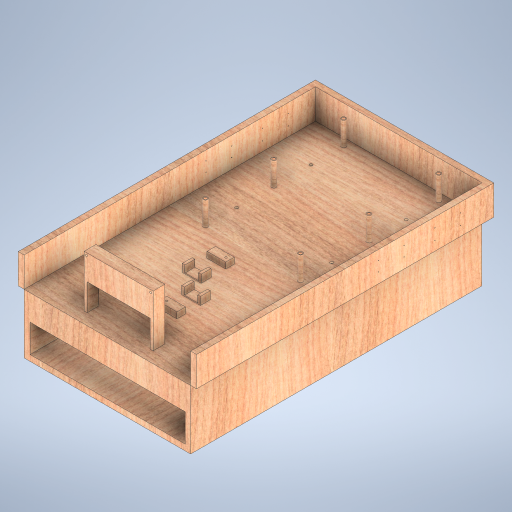
# Autodesk Inventor part: box
Saved by Autodesk Inventor 2024.3 (Build 283343000, 343)
## iProperties
Created: 2024-12-06
Part Number: box
Material: Wood (Birch)
Document SubType Name: Modeling
Designer: PRE 7730
Density: 0.55 g/cm^3
Appearance: Birch - Natural Polished
Author: PRE 7730
Autodesk Inventor part; units mm, degrees
ref_plane "YZ Plane" through (0, 0, 0) normal (1, 0, 0) x (0, 1, 0)
ref_plane "XZ Plane" through (0, 0, 0) normal (0, 1, 0) x (-1, 0, 0)
ref_plane "XY Plane" through (0, 0, 0) normal (0, 0, 1) x (1, 0, 0)
sketch "Sketch2" plane through (0, 0, 0) normal (0, 1, 0) x (-1, 0, 0)
  line L0 (14.4657, 20.7206) -> (-285.5343, 20.7206)
  line L1 (-285.5343, 20.7206) -> (-285.5343, -479.2794)
  line L2 (-285.5343, -479.2794) -> (14.4657, -479.2794)
  line L3 (14.4657, -479.2794) -> (14.4657, 20.7206)
  line L4 (-275.5343, 10.7206) -> (-275.5343, -469.2794)
  line L5 (-275.5343, -469.2794) -> (4.4657, -469.2794)
  line L6 (4.4657, -469.2794) -> (4.4657, 10.7206)
  line L7 (4.4657, 10.7206) -> (4.4657, 20.7206)
  line L8 (-275.5343, 10.7206) -> (-275.5343, 20.7206)
  point P0 (0, 0)
  dimension "d5" = 300
  dimension "d6" = 500
  dimension "d7" = 10
  constraints: 18 end point, 3 parallel, 3 perpendicular, 2 point on line, 1 horizontal, 2 other
  measures "d5" distance of L2.end L1.end
  measures "d6" distance of L1.end L0.end
  measures "d7" distance between parallel lines of L3 L6
extrude "Extrusion2" add sketch "Sketch2" against normal blind 100 contours L7 L6 L5 L4 L8 L0
extrude "Extrusion3" add sketch "Sketch2" along normal blind 50 contours L3 L2 L1 L0 L8 L4 L5 L6 L7
sketch "Sketch3" plane through (0, 0, 0) normal (0, 1, 0) x (1, 0, 0)
  point P0 (0, 0)
sketch "Sketch4" plane through (0, 0, 0) normal (0, 1, 0) x (1, 0, 0)
  line L0 (-4.4657, 469.2794) -> (-4.4657, -20.7206) projected
  line L1 (-4.4657, -20.7206) -> (275.5343, -20.7206) projected
  line L2 (275.5343, -20.7206) -> (275.5343, 469.2794) projected
  line L3 (275.5343, 469.2794) -> (-4.4657, 469.2794) projected
  line L4 (265.5343, 439.2794) -> (165.5343, 439.2794)
  line L5 (165.5343, 439.2794) -> (165.5343, 364.2794)
  line L6 (165.5343, 364.2794) -> (265.5343, 364.2794)
  line L7 (265.5343, 364.2794) -> (265.5343, 439.2794)
  line L8 (-4.4657, 469.2794) -> (275.5343, 469.2794)
  line L9 (-4.4657, 469.2794) -> (275.5343, 469.2794)
  line L10 (135.5343, 469.2794) -> (135.5343, 234.4175)
  line L11 (0, 339.2794) -> (275.5343, 339.2794)
  line L12 (5.5343, 439.2794) -> (105.5343, 439.2794)
  line L13 (105.5343, 439.2794) -> (105.5343, 364.2794)
  line L14 (105.5343, 364.2794) -> (5.5343, 364.2794)
  line L15 (5.5343, 364.2794) -> (5.5343, 439.2794)
  line L16 (265.5343, 239.2794) -> (165.5343, 239.2794)
  line L17 (165.5343, 239.2794) -> (165.5343, 314.2794)
  line L18 (165.5343, 314.2794) -> (265.5343, 314.2794)
  line L19 (265.5343, 314.2794) -> (265.5343, 239.2794)
  line L20 (5.5343, 239.2794) -> (105.5343, 239.2794)
  line L21 (105.5343, 239.2794) -> (105.5343, 314.2794)
  line L22 (105.5343, 314.2794) -> (5.5343, 314.2794)
  line L23 (5.5343, 314.2794) -> (5.5343, 239.2794)
  line L24 (135.5343, 79.3017) -> (167.0343, 79.3017)
  line L25 (167.0343, 79.3017) -> (167.0343, 64.8017)
  line L26 (167.0343, 64.8017) -> (135.5343, 64.8017)
  line L27 (135.5343, 64.8017) -> (135.5343, 79.3017)
  circle A0 centre (142.2843, 72.2017) radius 1.5
  line L28 (135.5343, 120.7409) -> (167.2853, 120.7409)
  line L29 (167.2853, 120.7409) -> (167.2853, 103.9909)
  line L30 (167.2853, 103.9909) -> (135.5343, 103.9909)
  line L31 (135.5343, 103.9909) -> (135.5343, 120.7409)
  line L32 (135.5343, 192.8569) -> (135.5343, 178.3569)
  line L33 (135.5343, 153.6678) -> (135.5343, 136.9178)
  line L34 (103.7833, 136.9178) -> (103.7833, 153.6678)
  line L35 (103.7833, 153.6678) -> (135.5343, 153.6678)
  circle A1 centre (128.7843, 185.4569) radius 1.5
  line L36 (135.5343, 178.3569) -> (104.0343, 178.3569)
  line L37 (104.0343, 178.3569) -> (104.0343, 192.8569)
  line L38 (104.0343, 192.8569) -> (135.5343, 192.8569)
  line L39 (135.5343, 136.9178) -> (103.7833, 136.9178)
  circle A2 centre (55.5343, 401.7794) radius 2.5
  circle A3 centre (215.5343, 401.7794) radius 2.5
  circle A4 centre (55.5343, 276.7794) radius 2.5
  circle A5 centre (215.5343, 276.7794) radius 2.5
  line L40 (275.5343, 469.2794) -> (275.5343, -20.7206) projected
  line L41 (-4.4657, -20.7206) -> (275.5343, -20.7206)
  line L42 (275.5343, -20.7206) -> (275.5343, -10.7206)
  line L43 (-4.4657, -10.7206) -> (-4.4657, -20.7206)
  line L44 (-4.4657, 469.2794) -> (-4.4657, -20.7206) projected
  line L45 (-4.4657, -20.7206) -> (275.5343, -20.7206) projected
  line L46 (275.5343, -20.7206) -> (275.5343, 469.2794) projected
  line L47 (275.5343, 469.2794) -> (-4.4657, 469.2794) projected
  line L48 (77.5343, 18.1016) -> (193.5343, 18.1016)
  line L49 (193.5343, 18.1016) -> (193.5343, -1.8984)
  line L50 (193.5343, -1.8984) -> (77.5343, -1.8984)
  line L51 (77.5343, -1.8984) -> (77.5343, 18.1016)
  circle A6 centre (55.5343, 456.7551) radius 3.75
  circle A7 centre (55.5343, 339.2794) radius 3.75
  circle A8 centre (55.5343, 224.2794) radius 3.75
  circle A9 centre (215.5343, 456.7551) radius 3.75
  circle A10 centre (215.5343, 339.2794) radius 3.75
  circle A11 centre (215.5343, 224.2794) radius 3.75
  circle A12 centre (55.5343, 456.7551) radius 2.5
  circle A13 centre (215.5343, 456.7551) radius 2.5
  circle A14 centre (215.5343, 339.2794) radius 2.5
  circle A15 centre (215.5343, 224.2794) radius 2.5
  circle A16 centre (55.5343, 224.2794) radius 2.5
  circle A17 centre (55.5343, 339.2794) radius 2.5
  point P0 (0, 0)
  point P1 (77.5343, 8.1016)
  dimension "d13" = 100
  dimension "d14" = 75
  dimension "d15" = 30
  dimension "d16" = 10
  dimension "d18" = 25
  dimension "d33" = 31.5
  dimension "d34" = 14.5
  dimension "d35" = 3
  dimension "d36" = 6.75
  dimension "d37" = 7.1
  dimension "d38" = 31.751
  dimension "d39" = 16.75
  dimension "d69" = 5
  dimension "d70" = 37.5
  dimension "d71" = 50
  dimension "d75" = 116
  dimension "d76" = 20
  dimension "d77" = 82
  dimension "d90" = 7.5
  dimension "d91" = 80
  dimension "d92" = 7.5
  dimension "d93" = 80
  dimension "d94" = 7.5
  dimension "d95" = 80
  dimension "d98" = 5
  dimension "d99" = 5
  dimension "d100" = 5
  dimension "d101" = 5
  dimension "d102" = 5
  dimension "d103" = 5
  constraints: 86 end point, 18 centre point, 18 symmetric about line, 9 parallel, 8 perpendicular, 6 coincident, 5 horizontal, 3 point on line, 2 midpoint, 1 vertical, 6 other
  measures "d13" distance of L6.end L5.end
  measures "d14" distance of L5.end L4.end
  measures "d15" distance between parallel lines of L4 L3
  measures "d16" distance between parallel lines of L2 L7
  measures "d18" distance between parallel lines of L11 L6
  measures "d33" distance of L25.end L26.end
  measures "d34" distance of L24.end L25.end
  measures "d35" diameter of A0
  measures "d36" distance from line of L27 A0.centre
  measures "d37" distance from line of L24 A0.centre
  measures "d38" distance of L29.end L30.end
  measures "d39" distance of L28.end L29.end
  measures "d69" diameter of A2
  measures "d70" distance from line of A2.centre L12
  measures "d71" distance from line of L15 A2.centre
  measures "d75" distance of L49.end L50.end
  measures "d76" distance of L48.end L49.end
  measures "d77" distance from line of L0 point (77.534, 8.102)
  measures "d90" diameter of A6
  measures "d91" distance from line of L10 A6.centre
  measures "d92" diameter of A7
  measures "d93" distance from line of L10 A7.centre
  measures "d94" diameter of A8
  measures "d95" distance from line of L10 A8.centre
  measures "d98" diameter of A12
  measures "d99" diameter of A13
  measures "d100" diameter of A14
  measures "d101" diameter of A15
  measures "d102" diameter of A16
  measures "d103" diameter of A17
extrude "Extrusion4" add sketch "Sketch4" along normal blind 10 contours L32 L36 L37 L38
sketch "Sketch5" plane through (-4.4657, -100, 20.7206) normal (0, 0, 1) x (1, 0, 0)
  line L0 (0, 100) -> (0, 0) projected
  line L1 (0, 67.0561) -> (280.9321, 67.0561)
  line L2 (280.9321, 67.0561) -> (280.9321, 0)
  line L3 (280.9321, 0) -> (0, 0)
  line L4 (0, 0) -> (0, 67.0561)
  line L5 (270.9321, 57.0561) -> (10, 57.0561)
  line L6 (10, 57.0561) -> (10, 10)
  line L7 (10, 10) -> (270.9321, 10)
  line L8 (270.9321, 10) -> (270.9321, 57.0561)
  point P0 (4.4657, 100)
  dimension "d24" = 10
  constraints: 16 end point, 4 perpendicular, 1 collinear, 1 horizontal, 1 point on line, 3 other
  measures "d24" distance between parallel lines of L1 L5
extrude "Extrusion5" cut sketch "Sketch5" against normal through all contours L8 L7 L6 L5
extrude "Extrusion6" add sketch "Sketch4" along normal blind 10 contours L33 L39 L34 L35
extrude "Extrusion7" add sketch "Sketch4" along normal blind 13 contours L28 L29 L30 L31 | L33 L39 L34 L35
extrude "Extrusion8" add sketch "Sketch4" along normal blind 10 contours L24 L25 L26 L27
sketch "Sketch6" plane through (0, 13, 0) normal (0, 1, 0) x (1, 0, 0)
  line L0 (104.0343, 192.8569) -> (135.5343, 192.8569) projected
  line L1 (135.5343, 192.8569) -> (135.5343, 178.3569) projected
  line L2 (135.5343, 178.3569) -> (104.0343, 178.3569) projected
  line L3 (104.0343, 178.3569) -> (104.0343, 192.8569) projected
  line L4 (-4.4657, 469.2794) -> (-4.4657, -20.7206) projected
  line L5 (-4.4657, -20.7206) -> (275.5343, -20.7206) projected
  line L6 (275.5343, -20.7206) -> (275.5343, 469.2794) projected
  line L7 (275.5343, 469.2794) -> (-4.4657, 469.2794) projected
  line L8 (103.7833, 153.6678) -> (135.5343, 153.6678) projected
  line L9 (135.5343, 153.6678) -> (135.5343, 136.9178) projected
  line L10 (135.5343, 136.9178) -> (103.7833, 136.9178) projected
  line L11 (103.7833, 136.9178) -> (103.7833, 153.6678) projected
  line L12 (135.5343, 103.9909) -> (135.5343, 120.7409) projected
  line L13 (135.5343, 120.7409) -> (167.2853, 120.7409) projected
  line L14 (167.2853, 120.7409) -> (167.2853, 103.9909) projected
  line L15 (167.2853, 103.9909) -> (135.5343, 103.9909) projected
  line L16 (135.5343, 64.8017) -> (135.5343, 79.3017) projected
  line L17 (135.5343, 79.3017) -> (167.0343, 79.3017) projected
  line L18 (167.0343, 79.3017) -> (167.0343, 64.8017) projected
  line L19 (167.0343, 64.8017) -> (135.5343, 64.8017) projected
  line L20 (103.7833, 153.6678) -> (135.5343, 153.6678)
  line L21 (135.5343, 153.6678) -> (135.5343, 136.9178)
  line L22 (135.5343, 136.9178) -> (103.7833, 136.9178)
  line L23 (103.7833, 136.9178) -> (103.7833, 153.6678)
  line L24 (108.4088, 153.6678) -> (108.4088, 136.9178)
  line L25 (103.7833, 153.6678) -> (135.5343, 153.6678) projected
  line L26 (130.9088, 153.6678) -> (130.9088, 136.9178)
  line L27 (135.5343, 120.7409) -> (167.2853, 120.7409)
  line L28 (167.2853, 120.7409) -> (167.2853, 103.9909)
  line L29 (167.2853, 103.9909) -> (135.5343, 103.9909)
  line L30 (135.5343, 103.9909) -> (135.5343, 120.7409)
  line L31 (135.5343, 120.7409) -> (167.2853, 120.7409) projected
  line L32 (140.1598, 120.7409) -> (140.1598, 103.9909)
  line L33 (162.6598, 120.7409) -> (162.6598, 103.9909)
  point P0 (0, 0)
  point P1 (135.5343, 112.3659)
  point P2 (140.1598, 112.3659)
  dimension "d46" = 22.5
  dimension "d47" = 4.6255
  dimension "d48" = 4.6255
  dimension "d49" = 22.5
  constraints: 24 end point, 8 point on line, 6 perpendicular, 4 parallel, 2 horizontal, 2 midpoint
  measures "d46" distance between parallel lines of L26 L24
  measures "d47" distance between parallel lines of L23 L24
  measures "d48" distance from line of point (135.534, 112.366) L32
  measures "d49" distance from line of point (140.16, 112.366) L33
extrude "Extrusion9" cut sketch "Sketch6" against normal blind 11.5 contours L8 L26 L10 L24 | L32 L13 L33 L15
sketch "Sketch7" plane through (-4.4657, 0, 20.7206) normal (1, 0, 0) x (0, 0, -1)
  line L0 (0, 0) -> (490, 0) projected
  line L1 (490, 50) -> (0, 50) projected
  line L2 (490, 0) -> (490, 50)
  line L3 (0, 0) -> (500, 0) projected
  line L4 (500, 0) -> (500, 50) projected
  line L5 (0, 50) -> (500, 50) projected
  line L6 (0, 0) -> (0, 50) projected
  line L7 (490, 0) -> (490, 50)
  line L8 (490, 50) -> (445, 50)
  line L9 (445, 50) -> (445, 35)
  line L10 (445, 35) -> (400, 35)
  line L11 (400, 35) -> (400, 15)
  line L12 (400, 15) -> (445, 15)
  line L13 (445, 15) -> (445, 35)
  line L14 (400, 35) -> (350, 35)
  line L15 (350, 35) -> (350, 15)
  line L16 (350, 15) -> (305, 15)
  line L17 (305, 15) -> (305, 35)
  line L18 (305, 35) -> (350, 35)
  circle A0 centre (444.165, 34.165) radius 0.5
  line L19 (445, 35) -> (422.5, 35)
  line L20 (422.5, 35) -> (422.5, 15)
  line L21 (445, 35) -> (445, 25)
  line L22 (445, 25) -> (400, 25)
  circle A1 centre (444.165, 15.835) radius 0.5
  circle A2 centre (400.835, 34.165) radius 0.5
  circle A3 centre (400.835, 15.835) radius 0.5
  line L23 (305, 15.835) -> (305, 25)
  line L24 (350, 15) -> (327.5, 15)
  line L25 (327.5, 15) -> (327.5, 35)
  line L26 (305, 15.835) -> (305, 25.835)
  line L27 (305, 25.835) -> (350, 25.835)
  circle A4 centre (349.165, 34.165) radius 0.5
  circle A5 centre (349.165, 17.505) radius 0.5
  circle A6 centre (305.835, 34.165) radius 0.5
  circle A7 centre (305.835, 17.505) radius 0.5
  point P0 (20.7206, 0)
  dimension "d52" = 45
  dimension "d53" = 15
  dimension "d54" = 45
  dimension "d55" = 20
  dimension "d56" = 50
  dimension "d57" = 20
  dimension "d58" = 45
  dimension "d59" = 1
  dimension "d60" = 0.835
  dimension "d61" = 0.835
  dimension "d63" = 10
  dimension "d64" = 1
  dimension "d65" = 0.835
  dimension "d66" = 0.835
  constraints: 44 end point, 9 perpendicular, 8 centre point, 7 midpoint, 6 symmetric about line, 5 point on line, 2 collinear, 1 horizontal, 1 vertical, 6 other
  measures "d52" distance of L1.start L8.end
  measures "d53" distance of L8.end L9.end
  measures "d54" distance of L9.end L10.end
  measures "d55" distance of L10.end L11.end
  measures "d56" distance of L10.end L14.end
  measures "d57" distance of L14.end L15.end
  measures "d58" distance of L15.end L16.end
  measures "d59" diameter of A0
  measures "d60" distance from line of L10 A0.centre
  measures "d61" distance from line of L13 A0.centre
  measures "d63" distance of L23.start L26.end
  measures "d64" diameter of A4
  measures "d65" distance from line of L15 A4.centre
  measures "d66" distance from line of L18 A4.centre
extrude "Extrusion10" cut sketch "Sketch7" along normal mid plane 1159.25 contours A0 | A1 | A2 | A3 | A4 | A5 | A6 | A7
extrude "Extrusion11" cut sketch "Sketch4" against normal blind 3 contours A2 | A3 | A4 | A5
extrude "Extrusion12" add sketch "Sketch4" along normal blind 87 contours L48 L49 L50 L51
sketch "Sketch8" plane through (77.5343, 0, 1.8984) normal (0, 0, 1) x (1, 0, 0)
  line L0 (0, 87) -> (116, 87)
  line L1 (0, 0) -> (0, 87) projected
  line L2 (0, 50) -> (116, 50)
  circle A0 centre (112, 83) radius 1.75
  circle A1 centre (4, 83) radius 1.75
  line L3 (0, 50) -> (116, 50)
  line L4 (116, 50) -> (116, 0)
  line L5 (116, 0) -> (0, 0)
  line L6 (0, 0) -> (0, 50)
  line L7 (111, 10) -> (111, 45)
  line L8 (111, 45) -> (5, 45)
  line L9 (5, 45) -> (5, 10)
  line L10 (5, 10) -> (5, 0.58)
  line L11 (111, 10) -> (111, 0)
  line L12 (5, 0.58) -> (5, 0)
  line L13 (-82, 0) -> (198, 0) projected
  line L14 (5, 0) -> (111, 0)
  point P0 (-77.5343, 0)
  point P1 (5, 0)
  dimension "d82" = 3.5
  dimension "d87" = 5
  constraints: 26 end point, 3 parallel, 3 perpendicular, 3 point on line, 2 centre point, 2 horizontal, 2 vertical, 1 collinear, 2 other
  measures "d82" diameter of A0
  measures "d87" distance between parallel lines of L4 L7
extrude "Extrusion13" cut sketch "Sketch8" against normal blind 20 contours A0 | A1
extrude "Extrusion14" cut sketch "Sketch8" against normal blind 20 contours L12 L10 L9 L8 L7 L11 L5
extrude "Extrusion16" add sketch "Sketch4" along normal blind 40 contours A7 L11 A17 | L11 A17 A7 | A10 L11 A14 | L11 A14 A10 | A6 | A8 | A9 | A11
sketch "Sketch9" plane through (193.5343, 87, -18.1016) normal (0, 0, -1) x (-1, 0, 0)
  line L0 (43, -0.9568) -> (73, -0.9568)
  line L1 (73, -0.9568) -> (73, -29.1877)
  line L2 (73, -29.1877) -> (43, -29.1877)
  line L3 (43, -29.1877) -> (43, -0.9568)
  line L4 (0, -87) -> (0, 0) projected
  line L5 (43, -15.0722) -> (73, -15.0722)
  circle A0 centre (47, -15.0722) radius 2
  circle A1 centre (69, -15.0722) radius 2
  point P0 (193.5343, -87)
  dimension "d106" = 30
  dimension "d107" = 43
  dimension "d108" = 4
  dimension "d109" = 4
  dimension "d110" = 4
  dimension "d111" = 4
  constraints: 10 end point, 2 centre point, 2 midpoint, 2 parallel, 2 point on line, 1 horizontal, 1 perpendicular
  measures "d106" distance of L1.end L2.end
  measures "d107" distance from line of L4 L5.start
  measures "d108" diameter of A0
  measures "d109" diameter of A1
  measures "d110" distance from line of L3 A0.centre
  measures "d111" distance from line of L1 A1.centre
extrude "Extrusion17" cut sketch "Sketch9" against normal blind 10 contours A0 L5 | L5 A0 | A1 L5 | L5 A1
body "Solid2"
